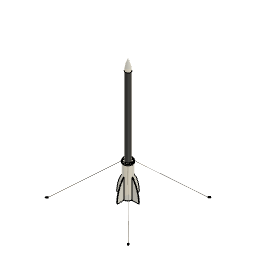
astra (Autodesk Fusion 360 design; units mm, degrees)
Autodesk Fusion 360 part; units mm, degrees
note: some values were not read from the file. Chosen so that the rebuilt part matches the saved one: which bodies a step acts on. Set by a fixed rule: which sketch regions a step uses.
sketch "Sketch1" plane through (0, 0, 0) normal (0, 1, 0) x (1, 0, 0)
sketch "Sketch2" plane through (0, 0, 0) normal (0, 0, 1) x (1, 0, 0)
  circle A0 centre (0, 0) radius 25
  circle A1 centre (0, 0) radius 24.5
  dimension "d1" = 50
  dimension "d2" = 49
  constraint coincident A0.centre A1.centre
  measures "d1" diameter of A0
  measures "d2" diameter of A1
extrude "Extrude1" add sketch "Sketch2" along normal blind 1000 makes body 1
sketch "Sketch3" plane through (0, 0, 0) normal (0, 1, 0) x (1, 0, 0)
sketch "Sketch4" plane through (0, 0, 0) normal (0, 0, 1) x (1, 0, 0)
  circle A0 centre (0, 0) radius 40
  circle A1 centre (0, 0) radius 39
  dimension "d5" = 80
  dimension "d6" = 78
  constraint coincident A0.centre A1.centre
  measures "d5" diameter of A0
  measures "d6" diameter of A1
extrude "Extrude2" add sketch "Sketch4" along normal blind 300 separate body makes body 2
sketch "Sketch5" plane through (0, 0, 0) normal (0, 0, 1) x (1, 0, 0)
sketch "Sketch6" plane through (0, 0, 0) normal (0, 0, 1) x (1, 0, 0)
  line L0 (0, -39) -> (-1, -39)
  line L1 (-1, -39) -> (-1, -25)
  line L2 (-1, -25) -> (0, -25)
  line L3 (0, -39) -> (1, -39)
  line L4 (1, -39) -> (1, -25)
  line L5 (1, -25) -> (0, -25)
  line L6 (39, 0) -> (39, -1)
  line L7 (39, -1) -> (25, -1)
  line L8 (25, -1) -> (25, 0)
  line L9 (39, 0) -> (39, 1)
  line L10 (39, 1) -> (25, 1)
  line L11 (25, 1) -> (25, 0)
  line L12 (0, 25) -> (1, 25)
  line L13 (1, 25) -> (1, 39)
  line L14 (1, 39) -> (0, 39)
  line L15 (0, 25) -> (-1, 25)
  line L16 (-1, 25) -> (-1, 39)
  line L17 (-1, 39) -> (0, 39)
  line L18 (-39, 0) -> (-39, -1)
  line L19 (-39, -1) -> (-25, -1)
  line L20 (-25, -1) -> (-25, 0)
  line L21 (-39, 0) -> (-39, 1)
  line L22 (-39, 1) -> (-25, 1)
  line L23 (-25, 1) -> (-25, 0)
  constraint horizontal L0
  constraint vertical L1
  constraint horizontal L2
  constraint horizontal L3
  constraint vertical L4
  constraint horizontal L5
  constraint vertical L6
  constraint horizontal L7
  constraint vertical L8
  constraint vertical L9
  constraint horizontal L10
  constraint vertical L11
  constraint horizontal L12
  constraint vertical L13
  constraint horizontal L14
  constraint horizontal L15
  constraint vertical L16
  constraint horizontal L17
  constraint vertical L18
  constraint horizontal L19
  constraint vertical L20
  constraint vertical L21
  constraint horizontal L22
  constraint vertical L23
extrude "Extrude3" cut sketch "Sketch6" along normal blind 2 bodies 2
extrude "Extrude4" cut sketch "Sketch6" along normal blind 2 bodies 2
extrude "Extrude5" cut sketch "Sketch6" along normal blind 2 contours L18 L19 L20 L21 L22 L23 bodies 2
extrude "Extrude6" add sketch "Sketch6" along normal blind 2 contours L6 L7 L8 L9 L10 L11 bodies 1 2
extrude "Extrude7" add sketch "Sketch6" along normal blind 2 separate body contours L12 L13 L14 L15 L16 L17 makes body 3
extrude "Extrude8" add sketch "Sketch6" along normal blind 2 separate body contours L18 L19 L20 L21 L22 L23 makes body 4
extrude "Extrude9" add sketch "Sketch6" along normal blind 2 separate body contours L0 L1 L2 L3 L4 L5 makes body 5
copy_body "CopyPasteBodies1" bodies 4 makes body 6
move_body "Move1" bodies 6 to x (1, 0, 0) y (0, 1, 0) z (0, 0, 1) at (0, 0, 260)
copy_body "CopyPasteBodies2" bodies 5 makes body 7
move_body "Move2" bodies 7 to x (1, 0, 0) y (0, 1, 0) z (0, 0, 1) at (0, 0, 260)
copy_body "CopyPasteBodies3" bodies 3 makes body 8
move_body "Move3" bodies 8 to x (1, 0, 0) y (0, 1, 0) z (0, 0, 1) at (0, 0, 260)
copy_body "CopyPasteBodies4" bodies 6 makes body 9
move_body "Move4" bodies 9 to x (1, 0, 0) y (0, 1, 0) z (0, 0, 1) at (64, 0, 0)
sketch "Sketch7" plane through (0, 0, 0) normal (0, 0, 1) x (1, 0, 0)
  circle A0 centre (-100, -50) radius 22.5
  circle A1 centre (-100, -50) radius 25
  circle A2 centre (-100, -50) radius 20
  line L0 (-150, -125) -> (-175, -125)
  arc A3 (-175, -125) -> (-150, -225) centre (77.618, -114.9705) ccw
  line L1 (-150, -225) -> (-150, -125)
  dimension "d24" = 45
  dimension "d25" = 50
  dimension "d26" = 40
  constraint concentric A0 A2
  constraint horizontal L0
  constraint perpendicular L0 L1
  measures "d24" diameter of A0
  measures "d25" diameter of A1
  measures "d26" diameter of A2
revolve "Revolve1" add sketch "Sketch7" angle 360 about axis through (-150, -225, 0) along (0, 1, 0) separate body contours L0 A3 L1 makes body 10
move_body "Move5" bodies 10 to x (1, 0, 0) y (0, 0, -1) z (0, 1, 0) at (0, 0, 875)
move_body "Move6" bodies 10 to x (1, 0, 0) y (0, 1, 0) z (0, 0, 1) at (150, 0, 0)
sketch "Sketch8" plane through (0, 0, 0) normal (0, 0, 1) x (1, 0, 0)
  line L0 (0, -250) -> (0, -190)
  line L1 (100, -190) -> (0, -190)
  line L2 (0, -190) -> (180, -190)
  arc A0 (0, -250) -> (180, -190) centre (-2.5, 57.5) ccw
  constraint vertical L0
  constraint perpendicular L0 L1
  constraint perpendicular L0 L2
extrude "Extrude10" add sketch "Sketch8" along normal blind 5 separate body makes body 11
move_body "Move7" bodies 11 to x (0, 0, 1) y (0, 1, 0) z (-1, 0, 0) at (0, 150, 0)
copy_body "CopyPasteBodies5" bodies 11 makes body 12
move_body "Move8" bodies 12 to x (0, -1, 0) y (1, 0, 0) z (0, 0, 1) at (0, -2.5, 0)
copy_body "CopyPasteBodies6" bodies 11 makes body 13
move_body "Move9" bodies 13 to x (-1, 0, 0) y (0, -1, 0) z (0, 0, 1) at (-2.5, -0.1, 0)
move_body "Move10" bodies 12 to x (1, 0, 0) y (0, 1, 0) z (0, 0, 1) at (0.4, 0, 0)
move_body "Move11" bodies 11 to x (1, 0, 0) y (0, 1, 0) z (0, 0, 1) at (2.5, 0.1, 0)
copy_body "CopyPasteBodies7" bodies 12 makes body 14
move_body "Move12" bodies 14 to x (-1, 0, 0) y (0, -1, 0) z (0, 0, 1) at (-1.2, 0, 0)
move_body "Move13" bodies 14 to x (1, 0, 0) y (0, 1, 0) z (0, 0, 1) at (1.5, 0, 0)
sketch "Sketch9" plane through (0, 0, 0) normal (0, 0, 1) x (1, 0, 0)
  circle A0 centre (150, 200) radius 40
  circle A1 centre (150, 200) radius 43
  dimension "d30" = 80
  dimension "d31" = 86
  constraint concentric A0 A1
  measures "d30" diameter of A0
  measures "d31" diameter of A1
extrude "Extrude11" add sketch "Sketch9" along normal blind 10 separate body makes body 15
move_body "Move14" bodies 15 to x (1, 0, 0) y (0, 1, 0) z (0, 0, 1) at (-150, -200, 280)
sketch "Sketch10" plane through (0, 0, 0) normal (0, 0, 1) x (1, 0, 0)
  circle A0 centre (175, 100) radius 5
  circle A1 centre (175, 100) radius 4.5
  circle A2 centre (175, 100) radius 4
  dimension "d41" = 10
  dimension "d42" = 9
  dimension "d43" = 8
  constraint concentric A0 A1
  constraint concentric A0 A2
  measures "d41" diameter of A0
  measures "d42" diameter of A1
  measures "d43" diameter of A2
extrude "Extrude14" add sketch "Sketch10" along normal blind 2.5 separate body contours A0 makes body 16
extrude "Extrude15" add sketch "Sketch10" along normal blind 2.5 separate body contours A2 makes body 17
combine "Combine1" operation add target body 17 tool bodies 16 makes body 18 at (179.9938, 99.7508, 1.6667)
combine "Combine2" operation add target body 18 tool bodies 17 makes body 19 at (178.6859, 101.5537, 1.6667)
combine "Combine3" operation add target body 19 tool bodies 18 makes body 20 at (179.9938, 99.7508, 1.6667)
move_body "Move15" bodies 20 19 to x (1, 0, 0) y (0, 1, 0) z (0, 0, 1) at (-90, 0, 0)
move_body "Move16" bodies 19 20 to x (1, 0, 0) y (0, 0, 1) z (0, -1, 0) at (0, 96, -96)
copy_body "CopyPasteBodies8" bodies 20 makes body 21
move_body "Move17" bodies 21 to x (1, 0, 0) y (0, 1, 0) z (0, 0, 1) at (0, 10, 0)
move_face "MoveFace1" by (0, 10, 0) 1 faces at (83.2053, 96, 4.5785) on bodies 19
move_body "Move18" bodies 21 19 20 to x (0.707107, 0.707107, 0) y (-0.707107, 0.707107, 0) z (0, 0, 1) at (43.0229, -96.6662, 281)
copy_body "CopyPasteBodies9" bodies 21 20 19 makes body 22 makes body 23 makes body 24
move_body "Move19" bodies 22 23 24 to x (1, 0, 0) y (0, 1, 0) z (0, 0, 1) at (-64.31, -69.3694, 0)
sketch "Sketch11" plane through (0, 0, 0) normal (0, 0, 1) x (1, 0, 0)
  line L0 (50, 50) -> (-50, -50)
  line L1 (-50, -50) -> (-50, 50)
  line L2 (-50, 50) -> (50, -50)
  line L3 (50, -50) -> (-50, -50)
  constraint vertical L1
  constraint perpendicular L0 L2
  constraint perpendicular L1 L3
combine "Combine4" operation add target body 20 tool bodies 21 19 makes body 25 at (32.8176, 40.6781, 284.0093) makes body 26 at (36.8386, 35.271, 284.2074)
move_body "Move20" bodies 20 26 25 to x (1, 0, 0) y (0, 1, 0) z (0, 0, 1) at (0, -1, 0)
move_body "Move21" bodies 24 23 22 to x (1, 0, 0) y (0, 1, 0) z (0, 0, 1) at (-1, 3, 0)
copy_body "CopyPasteBodies10" bodies 24 23 22 makes body 27 makes body 28 makes body 29
move_body "Move22" bodies 27 28 29 to x (0, 1, 0) y (-1, 0, 0) z (0, 0, 1) at (-64.6103, 65.3192, 0)
copy_body "CopyPasteBodies11" bodies 29 28 27 makes body 30 makes body 31 makes body 32
move_body "Move23" bodies 30 31 32 to x (1, 0, 0) y (0, 1, 0) z (0, 0, 1) at (65, -65, 0)
sketch "Sketch12" plane through (0, 0, 0) normal (0, 1, 0) x (1, 0, 0)
sketch "Sketch13" plane through (0, 0, 0) normal (0, 0, 1) x (1, 0, 0)
  circle A0 centre (25, 165) radius 1.25
  dimension "d51" = 2.5
  measures "d51" diameter of A0
extrude "Extrude17" add sketch "Sketch13" along normal blind 300 separate body makes body 33
move_body "Move26" bodies 33 to x (-0.819152, -0.564863, -0.099601) y (0.573576, -0.806707, -0.142244) z (0, -0.173648, 0.984808) at (-38.2436, 235.6431, 15.2907)
move_body "Move27" bodies 33 to x (0.707107, -0.707107, 0) y (0.707107, 0.707107, 0) z (0, 0, 1) at (-15.3946, 35.4662, 0)
move_face "MoveFace2" by (-0.307, -0.307, 2.462) 1 faces at (35.7092, 35.3378, 284.7241) on bodies 33
move_body "Move28" bodies 33 to x (1, 0, 0) y (0, 1, 0) z (0, 0, 1) at (5, 5, 0)
move_body "Move29" bodies 33 to x (0.707107, -0.696364, -0.122788) y (0.707107, 0.696364, 0.122788) z (0, -0.173648, 0.984808) at (-23.3901, 83.6468, 8.0045)
move_face "MoveFace3" by (-34.7296, -34.202, 193.9693) 1 faces at (34.0353, 34.1104, 290.985) on bodies 33
move_body "Move30" bodies 33 to x (0.984808, 0.157379, 0.073387) y (-0.173648, 0.892539, 0.416198) z (0, -0.422618, 0.906308) at (19.6854, 239.9744, -152.8923)
move_body "Move31" bodies 33 to x (0.866025, -0.5, 0) y (0.469846, 0.813798, 0.34202) z (-0.17101, -0.296198, 0.939693) at (-28.4059, -10.9362, -18.3514)
move_body "Move32" bodies 33 to x (1, 0, 0) y (0, 0.999229, 0.03926) z (0, -0.03926, 0.999229) at (0, -0.5545, 3.051)
move_body "Move33" bodies 33 to x (0.994522, -0.104528, 0) y (0.104528, 0.994522, 0) z (0, 0, 1) at (88.941, 117.8069, 20)
move_body "Move34" bodies 33 to x (1, 0, 0) y (0, 1, 0) z (0, 0, 1) at (0.2215, 0.0375, 2.2248)
move_face "MoveFace4" by (27.0961, 27.2763, -23.3838) 1 faces at (338.2331, 339.7868, 23.7501) on bodies 33
copy_body "CopyPasteBodies12" bodies 33 makes body 34
move_body "Move35" bodies 34 to x (-1, 0, 0) y (0, -1, 0) z (0, 0, 1) at (0.7735, 0.4247, 0)
copy_body "CopyPasteBodies13" bodies 34 makes body 35
move_body "Move36" bodies 35 to x (0, -1, 0) y (1, 0, 0) z (0, 0, 1) at (-2.8404, 0.3836, 0)
move_body "Move37" bodies 35 to x (1, 0, 0) y (0, 1, 0) z (0, 0, 1) at (2.9305, -0.4444, 1.455)
copy_body "CopyPasteBodies14" bodies 35 makes body 36
move_body "Move38" bodies 36 to x (-1, 0, 0) y (0, -1, 0) z (0, 0, 1) at (0.4092, -0.4092, 0)
sketch "Sketch14" plane through (0, 0, 0) normal (0, 0, 1) x (1, 0, 0)
  line L0 (200, 0) -> (210, 0)
  line L1 (210, 0) -> (210, -20)
  line L2 (210, -20) -> (200, -20)
  line L3 (200, -20) -> (200, 0)
  circle A0 centre (205, -2) radius 1.25
  line L4 (202.5, -5) -> (207.5, -5)
  line L5 (207.5, -5) -> (207.5, -15)
  line L6 (202.5, -15) -> (202.5, -5)
  line L7 (202.5, -15) -> (202.5, -17.5)
  line L8 (202.5, -17.5) -> (207.5, -17.5)
  line L9 (207.5, -17.5) -> (207.5, -15)
  dimension "d54" = 2.5
  constraint horizontal L0
  constraint vertical L1
  constraint horizontal L2
  constraint vertical L3
  constraint horizontal L4
  constraint vertical L5
  constraint vertical L6
  constraint parallel L6 L7
  constraint perpendicular L7 L8
  constraint perpendicular L8 L9
  measures "d54" diameter of A0
extrude "Extrude18" add sketch "Sketch14" along normal blind 2 separate body makes body 37
extrude "Extrude19" add sketch "Sketch14" against normal blind 3 separate body contours L4 L5 L6 L7 L8 L9 makes body 38
combine "Combine5" operation add target body 38 tool bodies 37
fillet "Fillet1" radius 2.5 1 faces at (204.1667, -9.1667, -3) on bodies 38
move_body "Move39" bodies 38 to x (0.707107, 0.707107, 0) y (-0.707107, 0.707107, 0) z (0, 0, 1) at (219.9758, -507.7269, 0)
copy_body "CopyPasteBodies15" bodies 38 makes body 39
move_body "Move40" bodies 39 to x (0, -1, 0) y (1, 0, 0) z (0, 0, 1) at (0.3448, -0.0506, 0)
copy_body "CopyPasteBodies16" bodies 39 makes body 40
move_body "Move41" bodies 40 to x (-1, 0, 0) y (0, -1, 0) z (0, 0, 1) at (0.3365, -0.2001, -0.0252)
copy_body "CopyPasteBodies17" bodies 38 makes body 41
move_body "Move42" bodies 41 to x (-1, 0, 0) y (0, -1, 0) z (0, 0, 1) at (0.213, -0.2841, 0)
move_body "Move43" bodies 41 to x (1, 0, 0) y (0, 1, 0) z (0, 0, 1) at (0.0939, -0.1409, 0)
sketch "Sketch15" plane through (0, 0, 0) normal (0, 0, 1) x (1, 0, 0)
  circle A0 centre (250, 50) radius 25
  circle A1 centre (250, 50) radius 1.25
  dimension "d61" = 50
  dimension "d62" = 2.5
  constraint concentric A0 A1
  measures "d61" diameter of A0
  measures "d62" diameter of A1
extrude "Extrude20" add sketch "Sketch15" along normal blind 2 separate body makes body 42
move_body "Move44" bodies 42 to x (1, 0, 0) y (0, 1, 0) z (0, 0, 1) at (-250, -50, 0)
sketch "Sketch16" plane through (0, 0, 0) normal (0, 0, 1) x (1, 0, 0)
  circle A0 centre (250, 100) radius 1.25
  circle A1 centre (250, 100) radius 1
  dimension "d65" = 2.5
  dimension "d66" = 2
  constraint concentric A0 A1
  measures "d65" diameter of A0
  measures "d66" diameter of A1
extrude "Extrude21" add sketch "Sketch16" along normal blind 4 separate body makes body 43
move_body "Move45" bodies 43 to x (1, 0, 0) y (0, 1, 0) z (0, 0, 1) at (-250, -100, 0)
move_body "Move46" bodies 43 to x (1, 0, 0) y (0, 1, 0) z (0, 0, 1) at (0, 0, -2)
move_face "MoveFace5" by (0, 0, -2) 1 faces at (0.8333, -79.9, 0) on bodies 11
move_face "MoveFace6" by (0, 0, -2) 1 faces at (79.9, 0.8333, 0) on bodies 14
move_face "MoveFace7" by (0, 0, -2) 1 faces at (-0.8333, 79.9, 0) on bodies 13
move_face "MoveFace8" by (0, 0, -2) 1 faces at (-79.6, -0.8333, 0) on bodies 12
